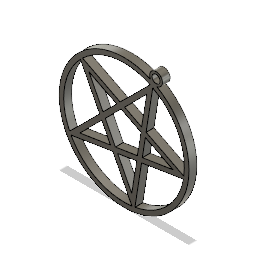
五角挂件 (Autodesk Fusion 360 design; units mm, degrees)
Autodesk Fusion 360 part; units mm, degrees
sketch "草图13" plane through (0, 0, 0) normal (0, 0, 1) x (1, 0, 0)
  circle A0 centre (-24, 17) radius 40.6099
  line L0 (-26.4265, 32.3206) -> (-7.8035, 50.9437)
  line L1 (-45.8508, 38.8508) -> (-28.657, 30.0901)
  line L2 (-23.616, 30.8886) -> (-9.9709, 44.5336)
  line L3 (-49.893, 44.2774) -> (-26.4265, 32.3206)
  line L4 (-9.9709, 44.5336) -> (-12.9896, 25.4742)
  line L5 (-23.616, 30.8886) -> (-12.9896, 25.4742)
  line L6 (-10.1791, 24.0421) -> (13.2874, 12.0854)
  line L7 (-6.059, 50.0549) -> (-10.1791, 24.0421)
  line L8 (-25.8465, 28.6581) -> (-13.4831, 22.3586)
  line L9 (-10.6725, 20.9266) -> (6.5212, 12.1659)
  line L10 (-10.6725, 20.9266) -> (-12.5382, 9.1472)
  line L11 (-13.0316, 6.0316) -> (-17.1517, -19.9811)
  line L12 (-13.4831, 22.3586) -> (-15.6537, 8.6537)
  line L13 (-16.1472, 5.5382) -> (-19.1659, -13.5212)
  line L14 (6.5212, 12.1659) -> (-12.5382, 9.1472)
  line L15 (12.9811, 10.1517) -> (-13.0316, 6.0316)
  line L16 (-27.9266, 3.6725) -> (-19.1659, -13.5212)
  line L17 (-15.6537, 8.6537) -> (-29.3586, 6.4831)
  line L18 (-32.4742, 5.9896) -> (-51.5336, 2.9709)
  line L19 (-31.0421, 3.1791) -> (-19.0854, -20.2874)
  line L20 (-16.1472, 5.5382) -> (-27.9266, 3.6725)
  line L21 (-31.0421, 3.1791) -> (-57.0549, -0.941)
  line L22 (-57.9437, 0.8035) -> (-39.3206, 19.4265)
  line L23 (-37.0901, 21.657) -> (-28.657, 30.0901)
  line L24 (-51.2774, 42.893) -> (-39.3206, 19.4265)
  line L25 (-37.8886, 16.616) -> (-32.4742, 5.9896)
  line L26 (-45.8508, 38.8508) -> (-37.0901, 21.657)
  line L27 (-35.6581, 18.8465) -> (-29.3586, 6.4831)
  line L28 (-51.5336, 2.9709) -> (-37.8886, 16.616)
  line L29 (-35.6581, 18.8465) -> (-25.8465, 28.6581)
  arc A1 (-7.8035, 50.9437) -> (-49.893, 44.2774) centre (-24, 17) ccw
  arc A2 (13.2874, 12.0854) -> (-6.059, 50.0549) centre (-24, 17) ccw
  arc A3 (-17.1517, -19.9811) -> (12.9811, 10.1517) centre (-24, 17) ccw
  arc A4 (-51.2774, 42.893) -> (-57.9437, 0.8035) centre (-24, 17) ccw
  arc A5 (-57.0549, -0.941) -> (-19.0854, -20.2874) centre (-24, 17) ccw
extrude "拉伸4" add sketch "草图13" along normal blind 5 makes body 1
sketch "草图14" plane through (0, 0, 0) normal (0, 0, 1) x (1, 0, 0)
  circle A0 centre (50, 15) radius 2.5
  circle A1 centre (50, 15) radius 4
  dimension "d36" = 5
  dimension "d37" = 8
  measures "d36" diameter of A0
  measures "d37" diameter of A1
extrude "拉伸5" add sketch "草图14" along normal blind 5 separate body makes body 2
move_body "移动2" bodies 2 to x (1, 0, 0) y (0, 1, 0) z (0, 0, 1) at (-75, 45, 0)
move_body "移动3" bodies 2 to x (1, 0, 0) y (0, 1, 0) z (0, 0, 1) at (21, -4, 0)
combine "合并5" operation add target body 2 tool bodies 1
sketch "草图11" plane through (0, 0, 0) normal (0, 0, 1) x (1, 0, 0)
  line L0 (-50, 25) -> (0, 25)
  line L1 (0, 25) -> (0, 5)
  line L2 (0, 5) -> (-50, 5)
  line L3 (-50, 5) -> (-50, 25)
  arc A0 (-50, 25) -> (-50, 5) centre (-51.9859, 15) ccw
  arc A1 (-50, 22.4346) -> (-50, 7.5654) centre (-51.9859, 15) ccw
extrude "拉伸2" [rolled back] along distance 3 taper angle 0
extrude "拉伸1" [rolled back] along distance 3 taper angle 0
sketch "草图12" plane through (0, 0, 3) normal (0, 0, 1) x (1, 0, 0)
  line L0 (-50, 5) -> (0, 5)
  line L1 (0, 5) -> (0, 25)
  line L2 (0, 25) -> (-50, 25)
  line L3 (-50, 25) -> (-50, 5)
  line L4 (-35, 12) -> (-16.2061, 12) construction
  line L5 (-16.2061, 12) -> (-16.2061, 22) construction
  line L6 (-16.2061, 22) -> (-35, 22) construction
  line L7 (-35, 22) -> (-35, 12) construction
extrude "拉伸3" [rolled back] along distance 2 taper angle 0
combine "合并4" [rolled back]
